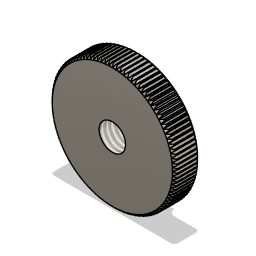
V Block assembly (Autodesk Fusion 360 archive; units mm, degrees)
design "Knurled Nut DIN 467 - M5 Steel 6 Plain"
description: Knurled Nut DIN 467 - M5
part number: DIN 467 - M5 Steel 6 Plain
Autodesk Fusion 360 part; units mm, degrees
sketch "Sketch1" plane through (0, 0, 0) normal (0, 1, 0) x (1, 0, 0)
  line L0 (0, 0) -> (0, -5)
  line L1 (-2.5, 0) -> (-2.5, -5)
  line L2 (-2.5, -5) -> (-10, -5)
  line L3 (-10, -5) -> (-10, -1)
  line L4 (-10, -1) -> (-5, -1)
  line L5 (-5, -1) -> (-5, 0)
  line L6 (-5, 0) -> (-2.5, 0)
  dimension "d195" = 5
  dimension "d196" = 4
  dimension "d197" = 20
  dimension "d198" = 5
  dimension "d199" = 10
  constraint coincident L0.start origin
  constraint vertical L0
  constraint parallel L0 L1
  constraint perpendicular L1 L2
  constraint perpendicular L2 L3
  constraint perpendicular L1 L4
  constraint perpendicular L4 L5
  constraint perpendicular L1 L6
  constraint coincident L0.end L2
  constraint coincident L0.start L6
  measures "d195" distance of L0.start L0.end
  measures "d196" distance of L2.end L3.end
revolve "Revolve1" add sketch "Sketch1" angle 360 about axis through (0, 0, 0) along (0, 0, 1)
chamfer "Chamfer4" distance 0.4 angle 45 2 edges at (-9.3233, 3.6162, 5) (-9.3233, 3.6162, 1) measured on face at (-9.9503, 0.9957, 3.6667) measured on face at (-8.2775, 0.7452, 1)
fillet "Fillet5" radius 1 1 edges at (-4.6616, 1.8081, 1)
sketch "Sketch22" plane through (0, 0, 5) normal (0, 0, 1) x (1, 0, 0)
  line L0 (-0.2309, 9.9973) -> (0, 9.5973)
  line L1 (0, 9.5973) -> (0.2309, 9.9973)
  line L2 (0, 0) -> (0, 10) construction
  circle A0 centre (0, 0) radius 2.5
  circle A1 centre (0, 0) radius 10
  dimension "d169" = 60
  dimension "d186" = 150
  dimension "d216" = 0.4
  constraint vertical L2
  constraint coincident L0.end L2
  constraint coincident L1.end A1
  constraint coincident L0.start A1
  constraint coincident L2.start A0.centre
  constraint coincident L2.end A1
  measures "d169" angle of L0 L1
  measures "d186" angle of L0 L2
  measures "d216" vertical distance of L0.end L1.end
extrude "Extrude11" cut sketch "Sketch22" against normal blind 5 contours L0 L1 A1 picked at (0, 9.8656)
pattern_circular "C-Pattern4" count 100 over 360 about axis through (0, 0, 1.75) along (0, 0, 1) of "Extrude11"
thread "Thread4" "ISO Metric profile 5.0 M5x0.8 6H" major diameter 5.12 minor diameter 4.234 pitch 0.8 angle 60 resizes the face on face at (-2.4969, 0.1246, 1.6667)
equation "adsk_maxdia = 20.00 mm"
equation "adsk_nomdia = 5.00 mm"
equation "adsk_nheig = 5.00 mm"
equation "d158 = adsk_chamheig"
equation "adsk_chamheig = 0.40 mm"
equation "d173 = -adsk_nheig"
equation "adsk_midrad = 1.00 mm"
equation "adsk_beardia = 10.00 mm"
equation "adsk_baseh = 4.00 mm"
equation "d195 = adsk_nheig"
equation "d196 = adsk_baseh"
equation "d197 = adsk_maxdia"
equation "d198 = adsk_nomdia"
equation "d199 = adsk_beardia"
equation "d203 = adsk_midrad"
equation "d214 = adsk_nheig"
equation "d216 = adsk_maxdia * 0.02"
